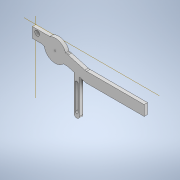
# Autodesk Inventor part: P6
Saved by Autodesk Inventor 2022 (Build 260153000, 153)
## iProperties
Created: 2022-11-21
Part Number: P6
Material: Genérico
Document SubType Name: Modeling
Designer: javie
Density: 1 g/cm^3
Appearance: Valor por defecto
Author: javie
Autodesk Inventor part; units mm, degrees
ref_plane "YZ Plane" through (0, 0, 0) normal (1, 0, 0) x (0, 1, 0)
ref_plane "XZ Plane" through (0, 0, 0) normal (0, 1, 0) x (-1, 0, 0)
ref_plane "XY Plane" through (0, 0, 0) normal (0, 0, 1) x (1, 0, 0)
sketch "Boceto1" plane through (0, 0, 0) normal (0, 0, 1) x (1, 0, 0)
  circle A0 centre (7, -5) radius 3.5
  arc A1 (66.7617, -38.7297) -> (62.7617, -38.7297) centre (64.7617, -38.7297) ccw
  line L0 (66.7617, -38.7297) -> (66.7617, -75.9094)
  arc A2 (62.7617, -75.9094) -> (66.7617, -75.9094) centre (64.7617, -75.9094) ccw
  line L1 (62.7617, -75.9094) -> (62.7617, -38.7297)
  line L2 (163.1909, -24.7137) -> (163.1909, -17.2137)
  line L3 (163.1909, -17.2137) -> (79.2209, -17.2137)
  arc A3 (76.5087, -16.8389) -> (79.2209, -17.2137) centre (79.2209, -7.2137) ccw
  line L4 (76.5087, -16.8389) -> (52.321, -10.0234)
  arc A4 (52.321, -10.0234) -> (50.4155, -9.6811) centre (49.6089, -19.6486) ccw
  arc A5 (48.4983, -9.3356) -> (50.4155, -9.6811) centre (51.2221, 0.2863) ccw
  arc A6 (17.4207, -16.6942) -> (45.0673, -24.7137) centre (33.1909, -13.9922) ccw
  line L5 (45.0673, -24.7137) -> (49.8402, -24.7137)
  arc A7 (52.5523, -25.0885) -> (49.8402, -24.7137) centre (49.8402, -34.7137) ccw
  line L6 (52.5523, -25.0885) -> (60.7617, -27.4017)
  line L7 (60.7617, -27.4017) -> (60.7617, -79.4017)
  arc A8 (60.7617, -79.4017) -> (68.7617, -79.4017) centre (64.7617, -79.6579) ccw
  line L8 (68.7617, -79.4017) -> (68.7617, -29.656)
  line L9 (68.7617, -29.656) -> (76.5087, -31.8389)
  arc A9 (76.5087, -31.8389) -> (79.2209, -32.2137) centre (79.2209, -22.2137) ccw
  line L10 (79.2209, -32.2137) -> (163.1909, -32.2137)
  line L11 (163.1909, -32.2137) -> (163.1909, -17.2137)
  line L12 (25.4308, 0) -> (0, 0)
  line L13 (0, 0) -> (0, -14.9941)
  line L14 (0, -14.9941) -> (11.843, -14.9941)
  arc A10 (17.4207, -16.6942) -> (11.843, -14.9941) centre (11.843, -24.9941) ccw
  arc A11 (48.4983, -9.3356) -> (25.4308, 0) centre (33.1909, -13.9922) ccw
  circle A12 centre (33.1909, -13.9922) radius 1
  point P0 (52.321, -10.0234)
  point P1 (50.4155, -9.6811)
  point P2 (48.4983, -9.3356)
  point P3 (11.843, -14.9941)
  point P4 (17.4207, -16.6942)
  point P5 (45.0673, -24.7137)
  point P6 (49.8402, -24.7137)
  point P7 (52.5523, -25.0885)
  point P8 (60.7617, -79.4017)
  point P9 (68.7617, -79.4017)
  point P10 (79.2209, -32.2137)
  dimension "d0" = 2
  constraints: 30 end point, 22 point on circle, 13 centre point, 1 coincident
  measures "d0" diameter of A12
extrude "Extrusión1" add sketch "Boceto1" along normal blind 5
